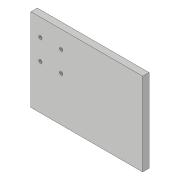
# Autodesk Inventor part: base1
Saved by Autodesk Inventor 2019 (Build 230136000, 136)
## iProperties
Created: 2019-10-12
Part Number: base1
Material: Generic
Document SubType Name: Modeling
Designer: Admin
Density: 1 g/cm^3
Appearance: Default
Author: Admin
Autodesk Inventor part; units mm, degrees
ref_plane "YZ Plane" through (0, 0, 0) normal (1, 0, 0) x (0, 1, 0)
ref_plane "XZ Plane" through (0, 0, 0) normal (0, 1, 0) x (-1, 0, 0)
ref_plane "XY Plane" through (0, 0, 0) normal (0, 0, 1) x (1, 0, 0)
sketch "Sketch1" plane through (0, 0, 0) normal (0, 0, 1) x (1, 0, 0)
  line L0 (0, 0) -> (350, 0)
  line L1 (350, 0) -> (350, 260)
  line L2 (350, 260) -> (0, 260)
  line L3 (0, 260) -> (0, 0)
  dimension "d0" = 350
  dimension "d1" = 260
  constraints: 8 end point, 2 parallel, 1 horizontal, 1 perpendicular
  measures "d0" distance of L2.end L1.end
  measures "d1" distance of L1.end L0.end
extrude "Extrusion1" add sketch "Sketch1" along normal blind 20
sketch "Sketch2" plane through (0, 0, 20) normal (0, 0, 1) x (1, 0, 0)
  line L0 (0, 0) -> (30, 0)
  line L1 (0, 0) -> (350, 0) projected
  line L2 (30, 0) -> (30, 260)
  dimension "d4" = 30
  constraints: 4 end point, 1 point on line
  measures "d4" distance of L0.start L0.end
sketch "Sketch3" plane through (0, 0, 20) normal (0, 0, 1) x (1, 0, 0)
  line L0 (0, 0) -> (0, 55)
  line L1 (0, 260) -> (0, 0) projected
  line L2 (0, 55) -> (31, 55)
  line L3 (0, 260) -> (0, 210)
  dimension "d5" = 55
  constraints: 6 end point, 2 point on line, 1 perpendicular
  measures "d5" distance of L0.start L0.end
sketch "Sketch4" plane through (0, 0, 20) normal (0, 0, 1) x (1, 0, 0)
  line L0 (350, 260) -> (0, 260) projected
  line L1 (0, 260) -> (0, 205)
  line L2 (0, 260) -> (0, 0) projected
  line L3 (0, 205) -> (29.7801, 205)
  line L4 (29.7801, 205) -> (94.7801, 205)
  line L5 (94.7801, 205) -> (94.7801, 140)
  line L6 (94.7801, 140) -> (29.7801, 140)
  circle A0 centre (29.7801, 205) radius 5
  circle A1 centre (29.7801, 140) radius 5
  circle A2 centre (94.7801, 140) radius 5
  circle A3 centre (94.7801, 205) radius 5
  dimension "d6" = 55
  dimension "d7" = 65
  dimension "d8" = 65
  dimension "d9" = 10
  dimension "d10" = 10
  dimension "d11" = 10
  dimension "d12" = 10
  constraints: 10 end point, 4 centre point, 4 coincident, 3 perpendicular, 2 point on line
  measures "d6" distance of L0.end L1.end
  measures "d7" distance of L3.end L4.end
  measures "d8" distance of L4.end L5.end
  measures "d9" diameter of A0
  measures "d10" diameter of A1
  measures "d11" diameter of A2
  measures "d12" diameter of A3
extrude "Extrusion2" cut sketch "Sketch4" against normal through all
body "Solid1"
